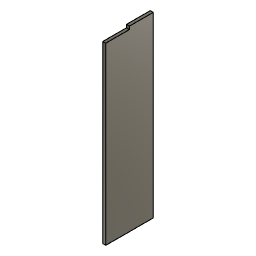
_ShelfSupport.d5eae4a0-9bc4-43bc-a936-d83c67e7b855 (Autodesk Fusion 360 design; units mm, degrees)
Autodesk Fusion 360 part; units mm, degrees
sketch "Sketch1" plane through (0, 0, 0) normal (1, 0, 0) x (0, 1, 0)
  line L0 (0, 0) -> (101.6, 0)
  line L1 (101.6, 0) -> (101.6, 381)
  line L2 (101.6, 381) -> (0, 381)
  line L3 (0, 381) -> (0, 0)
  line L4 (50.8, 381) -> (0, 381)
  line L5 (0, 381) -> (0, 374.65)
  line L6 (0, 374.65) -> (50.8, 374.65)
  line L7 (50.8, 374.65) -> (50.8, 381)
  dimension "d1" = 101.6
  dimension "d2" = 381
  dimension "d3" = 6.35
  dimension "d5" = 50.8
  constraint horizontal L0
  constraint vertical L1
  constraint horizontal L2
  constraint vertical L3
  constraint coincident L0.start L3.end
  constraint horizontal L4
  constraint vertical L5
  constraint horizontal L6
  constraint vertical L7
  constraint coincident L2 L4.start
  constraint collinear L3 L5
  measures "d1" distance of L0.start L0.end
  measures "d2" distance of L0.end L1.end
  measures "d3" distance of L2.end L5.end
  measures "d5" distance of L3 L7
extrude "Extrude1" add sketch "Sketch1" along normal blind 6.35 contours L0 L1 L2 L3 L6 L7
